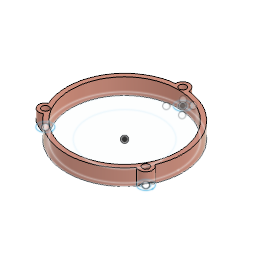
RingTop (Autodesk Fusion 360 design; units mm, degrees)
Autodesk Fusion 360 part; units mm, degrees
sketch "Sketch2" plane through (0, 0, 0) normal (0, 0, 1) x (1, 0, 0)
  circle A0 centre (0, 0) radius 35.9253
  circle A1 centre (0, 0) radius 22.5
  circle A2 centre (0, 35.9253) radius 2.15
  circle A3 centre (0, 35.9253) radius 4.15
  circle A4 centre (-31.1123, -17.9627) radius 2.15
  circle A5 centre (31.1123, -17.9627) radius 2.15
  circle A6 centre (0, 0) radius 33.1753
  line L0 (0, 40.0753) -> (0, 31.7753) construction
  line L1 (3.1373, 39.2901) -> (-4.8933, 30.6772) construction
  line L2 (-3.1373, 39.2901) -> (4.8933, 30.6772) construction
  circle A7 centre (-31.1123, -17.9627) radius 4.15
  circle A8 centre (31.1123, -17.9627) radius 4.15
  point P0 (0, 35.9253)
  dimension "d19" = 71.8507
  dimension "d21" = 45
  dimension "d22" = 4.3
  dimension "d23" = 2
  dimension "d25" = 360
  dimension "d29" = 66.3507
  constraint coincident A0.centre A1.centre
  constraint concentric A0 A1
  constraint coincident A0 P0
  constraint concentric A0 A6
  constraint coincident A3 L0.start
  constraint coincident A3 L0.end
  constraint vertical L0
  constraint coincident L1 P0
  constraint coincident L2 P0
  constraint coincident P0 A2.centre
  measures "d19" diameter of A0
  measures "d21" diameter of A1
  measures "d22" diameter of A2
  measures "d29" diameter of A6
extrude "main" add sketch "Sketch2" along normal blind 10 contours A0 A3 A6 A8 | A0 A2 A3 A6 | A0 A2 A3 | A0 A5 A8 | A0 A5 A6 A8 | A0 A3 A6 A7 | A0 A6 A7 A8 | A0 A4 A6 A7 | A0 A4 A7
sketch "Sketch4" plane through (0, 0, 0) normal (1, 0, 0) x (0, 1, 0)
  line L0 (0, 0) -> (35.9253, 0) construction
  line L1 (35.9253, 0) -> (52.3569, 16.4315)
  line L2 (35.9253, 0) -> (59.163, 0)
  line L3 (52.3569, 16.4315) -> (52.3569, 0)
  dimension "d69" = 35.9253
  dimension "d70" = 45
  constraint horizontal L0
  constraint coincident L0.start origin
  constraint horizontal L2
  constraint coincident L2 L3.end
  constraint perpendicular L2 L3
  measures "d69" distance of L0.start L0.end
  measures "d70" angle of L1 L2
extrude "Extrude8" cut sketch "Sketch4" along normal mid plane 20
pattern_circular "C-Pattern3" count 3 over 360 about axis through (0, 0, 1.75) along (0, 0, 1) of "Extrude8"
equation "gear_ratio = 6"
equation "gear_Ns = 12"
equation "gear_Nr = ( gear_ratio - 1 ) * gear_Ns"
equation "gear_OD = ( gear_Nr * diameter_scale * module ) + 8 mm"
equation "ring_width = 52 mm"
equation "m3_hole_thickness = 2 mm"
equation "m3_inserts = 4.3 mm"
equation "d19 = gear_OD"
equation "output_bearing_od = 47 mm"
equation "d21 = output_bearing_od - 2 mm"
equation "d22 = m3_inserts"
equation "d23 = m3_hole_thickness"
equation "d29 = gear_OD - wall_thickness + 1.5 mm"
equation "wall_thickness = 7 mm"
equation "d33 = height"
equation "height = 10 mm"
equation "module = 1"
equation "helix_angle = 20 deg"
equation "diameter_scale = ( 1 / cos(helix_angle) ) * 1 mm"
equation "d69 = gear_OD / 2"
